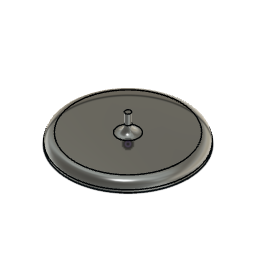
Base (Autodesk Fusion 360 design; units mm, degrees)
Autodesk Fusion 360 part; units mm, degrees
note: some values were not read from the file. Set by a fixed rule: which sketch regions a step uses.
sketch "Sketch1" plane through (0, 0, 0) normal (0, 0, 1) x (1, 0, 0)
  circle A0 centre (0, 0) radius 30
  dimension "d1" = 60
  constraint coincident A0.centre origin
  measures "d1" diameter of A0
extrude "Extrude3" add sketch "Sketch1" along normal blind 5.08
sketch "Sketch2" plane through (0, 0, 5.08) normal (0, 0, 1) x (-1, 0, 0)
  circle A0 centre (0, 0) radius 30
  circle A1 centre (0, 0) radius 1.35
  dimension "d11" = 2.7
  constraint coincident A0.centre A1.centre
  measures "d11" diameter of A1
fillet "Fillet2" radius 3.81 1 edges at (-27.9698, -10.8485, 5.08)
extrude "Extrude4" add sketch "Sketch2" along normal blind 8.89 contours A1
fillet "Fillet3" radius 3.81 1 edges at (1.2586, -0.4882, 5.08)
